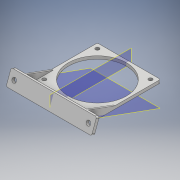
# Autodesk Inventor part: Eletronica - FanPlaca
Saved by Autodesk Inventor 2017 (Build 210142000, 142)
## iProperties
Created: 2020-11-08
Part Number: Eletronica - FanPlaca
Material: Generic
Document SubType Name: Modeling
Designer: ale
Density: 1 g/cm^3
Appearance: Default
Author: ale
Autodesk Inventor part; units mm, degrees
ref_plane "YZ Plane" through (0, 0, 0) normal (1, 0, 0) x (0, 1, 0)
ref_plane "XZ Plane" through (0, 0, 0) normal (0, 1, 0) x (-1, 0, 0)
ref_plane "XY Plane" through (0, 0, 0) normal (0, 0, 1) x (1, 0, 0)
sketch "Sketch1" plane through (0, 0, 0) normal (0, 0, 1) x (1, 0, 0)
  line L0 (-35.75, 35.75) -> (35.75, -35.75) construction
  line L1 (35.75, 35.75) -> (-35.75, -35.75) construction
  line L2 (-42.5, 42.5) -> (42.5, 42.5)
  line L3 (42.5, 42.5) -> (42.5, -42.5)
  line L4 (42.5, -42.5) -> (-42.5, -42.5)
  line L5 (-42.5, -42.5) -> (-42.5, 42.5)
  line L6 (-42.5, 42.5) -> (42.5, -42.5) construction
  line L7 (42.5, 42.5) -> (-42.5, -42.5) construction
  circle A0 centre (-35.75, 35.75) radius 2.5
  circle A1 centre (35.75, 35.75) radius 2.5
  circle A2 centre (-35.75, -35.75) radius 2.5
  circle A3 centre (35.75, -35.75) radius 2.5
  circle A4 centre (0, 0) radius 39
  dimension "d0" = 71.5
  dimension "d1" = 71.5
  dimension "d2" = 85
  dimension "d3" = 85
  dimension "d4" = 5
  dimension "d5" = 5
  dimension "d6" = 5
  dimension "d7" = 5
  dimension "d8" = 78
  constraints: 16 end point, 5 centre point, 5 coincident, 4 midpoint, 2 parallel, 1 horizontal, 1 perpendicular
  measures "d0" distance of L0.end L1.end
  measures "d1" distance of L1.start L0.end
  measures "d2" distance of L3.end L4.end
  measures "d3" distance of L2.end L3.end
  measures "d4" diameter of A0
  measures "d5" diameter of A1
  measures "d6" diameter of A2
  measures "d7" diameter of A3
  measures "d8" diameter of A4
extrude "Extrusion1" add sketch "Sketch1" along normal blind 4
ref_plane "Work Plane2" through (42.5, -42.5, 4) normal (0, -0.342, -0.9397) x (1, 0, 0)
sketch "Sketch4" plane through (42.5, -42.5, 4) normal (0, -0.342, -0.9397) x (1, 0, 0)
  line L0 (-85, 0) -> (0, 0) projected
  line L1 (0, 0) -> (-85, 0)
  line L2 (-85, 0) -> (-85, 16)
  line L3 (-85, 16) -> (0, 16)
  line L4 (0, 16) -> (0, 0)
  point P0 (-42.5, -41.305)
  dimension "d15" = 16
  constraints: 8 end point, 2 parallel, 1 horizontal, 1 perpendicular
  measures "d15" distance of L1.end L2.end
extrude "Extrusion2" add sketch "Sketch4" along normal blind 4
sketch "Sketch5" plane through (42.5, -57.5351, 9.4723) normal (1, 0, 0) x (0, -0.342, -0.9397)
  line L0 (0, 0) -> (0, 16) projected
  line L1 (3.7588, 17.3681) -> (0, 16) projected
  line L2 (0, 16) -> (3.7588, 17.3681)
  line L3 (4, 16) -> (4, 0) projected
  line L4 (3.7588, 17.3681) -> (4, 16)
  line L5 (4, 16) -> (0, 16)
  point P0 (-10.7771, 57.305)
  constraints: 6 end point, 1 collinear, 1 perpendicular
extrude "Extrusion3" add sketch "Sketch5" against normal blind 85
sketch "Sketch6" plane through (-42.5, -57.5351, 9.4723) normal (0, -0.9397, 0.342) x (1, 0, 0)
  line L0 (85, 0) -> (85, -4) projected
  line L1 (85, -4) -> (0, 0)
  line L2 (100, -12) -> (-15, -12)
  line L3 (-15, -12) -> (-15, 8)
  line L4 (-15, 8) -> (100, 8)
  line L5 (100, 8) -> (100, -12)
  line L6 (100, -12) -> (-15, 8) construction
  line L7 (-15, -12) -> (100, 8) construction
  circle A0 centre (92.5, -2) radius 3
  line L8 (42.5, 8) -> (42.5, -12)
  circle A1 centre (-7.5, -2) radius 3
  point P0 (42.5, -2)
  dimension "d20" = 115
  dimension "d21" = 20
  dimension "d22" = 6
  dimension "d23" = 7.5
  constraints: 16 end point, 5 midpoint, 2 centre point, 2 parallel, 1 horizontal, 1 perpendicular, 1 symmetric about line, 1 other
  measures "d20" distance of L3.end L4.end
  measures "d21" distance of L2.end L3.end
  measures "d22" diameter of A0
  measures "d23" distance from line of A0.centre L5
extrude "Extrusion4" add sketch "Sketch6" along normal blind 4
fillet "Fillet1" radius 2 6 edges at (57.5, -63.5187, -1.1199) (-57.5, -63.5187, -1.1199) (-57.5, -56.6783, 17.6739) (57.5, -56.6783, 17.6739) (42.5, 42.5, 2) (-42.5, 42.5, 2)
sketch "Sketch8" plane through (-42.5, -57.5351, 9.4723) normal (0, 0.9397, -0.342) x (1, 0, 0)
  line L0 (0, 0) -> (2, 0)
  line L1 (2, 0) -> (2, -8)
  line L2 (2, -8) -> (0, -8)
  line L3 (0, -8) -> (0, 0)
  point P0 (42.5, -10.7771)
  dimension "d33" = 2
  dimension "d34" = 8
  constraints: 8 end point, 2 parallel, 1 horizontal, 1 perpendicular
  measures "d33" distance of L1.end L2.end
  measures "d34" distance of L0.end L1.end
extrude "Extrusion6" add sketch "Sketch8" along normal up to surface surface through (0, 0, 4) normal (0, 0, 1)
ref_plane "Work Plane3" through (0, -42.5, 0) normal (-1, 0, 0) x (0, 0, 1)
mirror "Mirror1" about plane through (0, -42.5, 0) normal (-1, 0, 0) of "Extrusion6"
body "Solid1"
